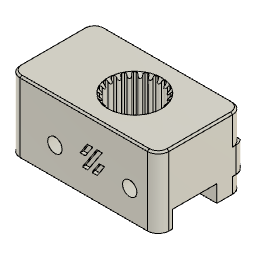
nozzle_probe_ldo (Autodesk Fusion 360 design; units mm, degrees)
Autodesk Fusion 360 part; units mm, degrees
sketch "Sketch1" plane through (0, 0, 0) normal (0, 0, 1) x (1, 0, 0)
  line L0 (17.5, 10) -> (-17.5, 10)
  line L1 (-17.5, 10) -> (-17.5, -10)
  line L2 (-17.5, -10) -> (17.5, -10)
  line L3 (17.5, -10) -> (17.5, 10)
  line L4 (17.5, 10) -> (-17.5, -10) construction
  line L5 (-17.5, 10) -> (17.5, -10) construction
  dimension "d5" = 35
  dimension "d6" = 20
  constraint horizontal L0
  constraint perpendicular L0 L1
  constraint parallel L0 L2
  constraint parallel L1 L3
  constraint coincident L4 origin
  constraint coincident L5 origin
  measures "d5" distance of L0.start L0.end
  measures "d6" distance of L0.start L2.end
extrude "Extrude1" add sketch "Sketch1" against normal blind 16.6
sketch "Sketch2" plane through (0, 0, 0) normal (0, 0, 1) x (-1, 0, 0)
  line L0 (-17.5, 10) -> (-17.5, -10)
  line L1 (-17.5, -10) -> (17.5, -10)
  line L2 (17.5, -10) -> (17.5, 10)
  line L3 (17.5, 10) -> (-17.5, 10)
  circle A0 centre (0, 0) radius 7.61 construction
  arc A1 (5.0953, -3.0231) -> (4.4497, -3.9118) centre (4.7489, -3.4503) ccw construction
  arc A2 (5.0953, -3.0231) -> (5.3358, -2.9768) centre (5.1961, -2.8988) ccw construction
  arc A3 (5.3358, -2.9768) -> (5.5446, -2.5671) centre (0, 0) ccw construction
  arc A4 (5.5446, -2.5671) -> (5.4407, -2.3453) centre (5.3994, -2.4999) ccw construction
  arc A5 (5.7801, -1.3006) -> (5.4407, -2.3453) centre (5.5827, -1.8139) ccw construction
  arc A6 (5.7801, -1.3006) -> (5.9945, -1.1822) centre (5.8376, -1.1512) ccw construction
  arc A7 (5.9945, -1.1822) -> (6.0665, -0.7281) centre (0, 0) ccw construction
  arc A8 (6.0665, -0.7281) -> (5.8991, -0.5492) centre (5.9076, -0.709) ccw construction
  arc A9 (5.8991, 0.5492) -> (5.8991, -0.5492) centre (5.87, 0) ccw construction
  arc A10 (5.8991, 0.5492) -> (6.0665, 0.7281) centre (5.9076, 0.709) ccw construction
  arc A11 (6.0665, 0.7281) -> (5.9945, 1.1822) centre (0, 0) ccw construction
  arc A12 (5.9945, 1.1822) -> (5.7801, 1.3006) centre (5.8376, 1.1512) ccw construction
  arc A13 (5.4407, 2.3453) -> (5.7801, 1.3006) centre (5.5827, 1.8139) ccw construction
  arc A14 (5.4407, 2.3453) -> (5.5446, 2.5671) centre (5.3994, 2.4999) ccw construction
  arc A15 (5.5446, 2.5671) -> (5.3358, 2.9768) centre (0, 0) ccw construction
  arc A16 (5.3358, 2.9768) -> (5.0953, 3.0231) centre (5.1961, 2.8988) ccw construction
  arc A17 (4.4497, 3.9118) -> (5.0953, 3.0231) centre (4.7489, 3.4503) ccw construction
  arc A18 (4.4497, 3.9118) -> (4.4799, 4.1548) centre (4.3626, 4.046) ccw construction
  arc A19 (4.4799, 4.1548) -> (4.1548, 4.4799) centre (0, 0) ccw construction
  arc A20 (4.1548, 4.4799) -> (3.9118, 4.4497) centre (4.046, 4.3626) ccw construction
  arc A21 (3.0231, 5.0953) -> (3.9118, 4.4497) centre (3.4503, 4.7489) ccw construction
  arc A22 (3.0231, 5.0953) -> (2.9768, 5.3358) centre (2.8988, 5.1961) ccw construction
  arc A23 (2.9768, 5.3358) -> (2.5671, 5.5446) centre (0, 0) ccw construction
  arc A24 (2.5671, 5.5446) -> (2.3453, 5.4407) centre (2.4999, 5.3994) ccw construction
  arc A25 (1.3006, 5.7801) -> (2.3453, 5.4407) centre (1.8139, 5.5827) ccw construction
  arc A26 (1.3006, 5.7801) -> (1.1822, 5.9945) centre (1.1512, 5.8376) ccw construction
  arc A27 (1.1822, 5.9945) -> (0.7281, 6.0665) centre (0, 0) ccw construction
  arc A28 (0.7281, 6.0665) -> (0.5492, 5.8991) centre (0.709, 5.9076) ccw construction
  arc A29 (-0.5492, 5.8991) -> (0.5492, 5.8991) centre (0, 5.87) ccw construction
  arc A30 (-0.5492, 5.8991) -> (-0.7281, 6.0665) centre (-0.709, 5.9076) ccw construction
  arc A31 (-0.7281, 6.0665) -> (-1.1822, 5.9945) centre (0, 0) ccw construction
  arc A32 (-1.1822, 5.9945) -> (-1.3006, 5.7801) centre (-1.1512, 5.8376) ccw construction
  arc A33 (-2.3453, 5.4407) -> (-1.3006, 5.7801) centre (-1.8139, 5.5827) ccw construction
  arc A34 (-2.3453, 5.4407) -> (-2.5671, 5.5446) centre (-2.4999, 5.3994) ccw construction
  arc A35 (-2.5671, 5.5446) -> (-2.9768, 5.3358) centre (0, 0) ccw construction
  arc A36 (-2.9768, 5.3358) -> (-3.0231, 5.0953) centre (-2.8988, 5.1961) ccw construction
  arc A37 (-3.9118, 4.4497) -> (-3.0231, 5.0953) centre (-3.4503, 4.7489) ccw construction
  arc A38 (-3.9118, 4.4497) -> (-4.1548, 4.4799) centre (-4.046, 4.3626) ccw construction
  arc A39 (-4.1548, 4.4799) -> (-4.4799, 4.1548) centre (0, 0) ccw construction
  arc A40 (-4.4799, 4.1548) -> (-4.4497, 3.9118) centre (-4.3626, 4.046) ccw construction
  arc A41 (-5.0953, 3.0231) -> (-4.4497, 3.9118) centre (-4.7489, 3.4503) ccw construction
  arc A42 (-5.0953, 3.0231) -> (-5.3358, 2.9768) centre (-5.1961, 2.8988) ccw construction
  arc A43 (-5.3358, 2.9768) -> (-5.5446, 2.5671) centre (0, 0) ccw construction
  arc A44 (-5.5446, 2.5671) -> (-5.4407, 2.3453) centre (-5.3994, 2.4999) ccw construction
  arc A45 (-5.7801, 1.3006) -> (-5.4407, 2.3453) centre (-5.5827, 1.8139) ccw construction
  arc A46 (-5.7801, 1.3006) -> (-5.9945, 1.1822) centre (-5.8376, 1.1512) ccw construction
  arc A47 (-5.9945, 1.1822) -> (-6.0665, 0.7281) centre (0, 0) ccw construction
  arc A48 (-6.0665, 0.7281) -> (-5.8991, 0.5492) centre (-5.9076, 0.709) ccw construction
  arc A49 (-5.8991, -0.5492) -> (-5.8991, 0.5492) centre (-5.87, 0) ccw construction
  arc A50 (-5.8991, -0.5492) -> (-6.0665, -0.7281) centre (-5.9076, -0.709) ccw construction
  arc A51 (-6.0665, -0.7281) -> (-5.9945, -1.1822) centre (0, 0) ccw construction
  arc A52 (-5.9945, -1.1822) -> (-5.7801, -1.3006) centre (-5.8376, -1.1512) ccw construction
  arc A53 (-5.4407, -2.3453) -> (-5.7801, -1.3006) centre (-5.5827, -1.8139) ccw construction
  arc A54 (-5.4407, -2.3453) -> (-5.5446, -2.5671) centre (-5.3994, -2.4999) ccw construction
  arc A55 (-5.5446, -2.5671) -> (-5.3358, -2.9768) centre (0, 0) ccw construction
  arc A56 (-5.3358, -2.9768) -> (-5.0953, -3.0231) centre (-5.1961, -2.8988) ccw construction
  arc A57 (-4.4497, -3.9118) -> (-5.0953, -3.0231) centre (-4.7489, -3.4503) ccw construction
  arc A58 (-4.4497, -3.9118) -> (-4.4799, -4.1548) centre (-4.3626, -4.046) ccw construction
  arc A59 (-4.4799, -4.1548) -> (-4.1548, -4.4799) centre (0, 0) ccw construction
  arc A60 (-4.1548, -4.4799) -> (-3.9118, -4.4497) centre (-4.046, -4.3626) ccw construction
  arc A61 (-3.0231, -5.0953) -> (-3.9118, -4.4497) centre (-3.4503, -4.7489) ccw construction
  arc A62 (-3.0231, -5.0953) -> (-2.9768, -5.3358) centre (-2.8988, -5.1961) ccw construction
  arc A63 (-2.9768, -5.3358) -> (-2.5671, -5.5446) centre (0, 0) ccw construction
  arc A64 (-2.5671, -5.5446) -> (-2.3453, -5.4407) centre (-2.4999, -5.3994) ccw construction
  arc A65 (-1.3006, -5.7801) -> (-2.3453, -5.4407) centre (-1.8139, -5.5827) ccw construction
  arc A66 (-1.3006, -5.7801) -> (-1.1822, -5.9945) centre (-1.1512, -5.8376) ccw construction
  arc A67 (-1.1822, -5.9945) -> (-0.7281, -6.0665) centre (0, 0) ccw construction
  arc A68 (-0.7281, -6.0665) -> (-0.5492, -5.8991) centre (-0.709, -5.9076) ccw construction
  arc A69 (0.5492, -5.8991) -> (-0.5492, -5.8991) centre (0, -5.87) ccw construction
  arc A70 (0.5492, -5.8991) -> (0.7281, -6.0665) centre (0.709, -5.9076) ccw construction
  arc A71 (0.7281, -6.0665) -> (1.1822, -5.9945) centre (0, 0) ccw construction
  arc A72 (1.1822, -5.9945) -> (1.3006, -5.7801) centre (1.1512, -5.8376) ccw construction
  arc A73 (2.3453, -5.4407) -> (1.3006, -5.7801) centre (1.8139, -5.5827) ccw construction
  arc A74 (2.3453, -5.4407) -> (2.5671, -5.5446) centre (2.4999, -5.3994) ccw construction
  arc A75 (2.5671, -5.5446) -> (2.9768, -5.3358) centre (0, 0) ccw construction
  arc A76 (2.9768, -5.3358) -> (3.0231, -5.0953) centre (2.8988, -5.1961) ccw construction
  arc A77 (3.9118, -4.4497) -> (3.0231, -5.0953) centre (3.4503, -4.7489) ccw construction
  arc A78 (3.9118, -4.4497) -> (4.1548, -4.4799) centre (4.046, -4.3626) ccw construction
  arc A79 (4.1548, -4.4799) -> (4.4799, -4.1548) centre (0, 0) ccw construction
  arc A80 (4.4799, -4.1548) -> (4.4497, -3.9118) centre (4.3626, -4.046) ccw construction
  arc A81 (-2.6301, -5.6807) -> (-2.2004, -5.4794) centre (-2.4999, -5.3994) ccw
  arc A82 (-1.4406, -5.7263) -> (-2.2004, -5.4794) centre (-1.8139, -5.5827) ccw
  arc A83 (-1.4406, -5.7263) -> (-1.2112, -6.1417) centre (-1.1512, -5.8376) ccw
  arc A84 (-1.2112, -6.1417) -> (-0.7459, -6.2154) centre (0, 0) ccw
  arc A85 (-0.7459, -6.2154) -> (-0.3994, -5.8912) centre (-0.709, -5.9076) ccw
  arc A86 (0.3994, -5.8912) -> (-0.3994, -5.8912) centre (0, -5.87) ccw
  arc A87 (0.3994, -5.8912) -> (0.7459, -6.2154) centre (0.709, -5.9076) ccw
  arc A88 (0.7459, -6.2154) -> (1.2112, -6.1417) centre (0, 0) ccw
  arc A89 (1.2112, -6.1417) -> (1.4406, -5.7263) centre (1.1512, -5.8376) ccw
  arc A90 (2.2004, -5.4794) -> (1.4406, -5.7263) centre (1.8139, -5.5827) ccw
  arc A91 (2.2004, -5.4794) -> (2.6301, -5.6807) centre (2.4999, -5.3994) ccw
  arc A92 (2.6301, -5.6807) -> (3.0498, -5.4668) centre (0, 0) ccw
  arc A93 (3.0498, -5.4668) -> (3.1396, -5.0009) centre (2.8988, -5.1961) ccw
  arc A94 (3.7859, -4.5313) -> (3.1396, -5.0009) centre (3.4503, -4.7489) ccw
  arc A95 (3.7859, -4.5313) -> (4.2568, -4.5899) centre (4.046, -4.3626) ccw
  arc A96 (4.2568, -4.5899) -> (4.5899, -4.2568) centre (0, 0) ccw
  arc A97 (4.5899, -4.2568) -> (4.5313, -3.7859) centre (4.3626, -4.046) ccw
  arc A98 (5.0009, -3.1396) -> (4.5313, -3.7859) centre (4.7489, -3.4503) ccw
  arc A99 (5.0009, -3.1396) -> (5.4668, -3.0498) centre (5.1961, -2.8988) ccw
  arc A100 (5.4668, -3.0498) -> (5.6807, -2.6301) centre (0, 0) ccw
  arc A101 (5.6807, -2.6301) -> (5.4794, -2.2004) centre (5.3994, -2.4999) ccw
  arc A102 (5.7263, -1.4406) -> (5.4794, -2.2004) centre (5.5827, -1.8139) ccw
  arc A103 (5.7263, -1.4406) -> (6.1417, -1.2112) centre (5.8376, -1.1512) ccw
  arc A104 (6.1417, -1.2112) -> (6.2154, -0.7459) centre (0, 0) ccw
  arc A105 (6.2154, -0.7459) -> (5.8912, -0.3994) centre (5.9076, -0.709) ccw
  arc A106 (5.8912, 0.3994) -> (5.8912, -0.3994) centre (5.87, 0) ccw
  arc A107 (5.8912, 0.3994) -> (6.2154, 0.7459) centre (5.9076, 0.709) ccw
  arc A108 (6.2154, 0.7459) -> (6.1417, 1.2112) centre (0, 0) ccw
  arc A109 (6.1417, 1.2112) -> (5.7263, 1.4406) centre (5.8376, 1.1512) ccw
  arc A110 (5.4794, 2.2004) -> (5.7263, 1.4406) centre (5.5827, 1.8139) ccw
  arc A111 (5.4794, 2.2004) -> (5.6807, 2.6301) centre (5.3994, 2.4999) ccw
  arc A112 (5.6807, 2.6301) -> (5.4668, 3.0498) centre (0, 0) ccw
  arc A113 (5.4668, 3.0498) -> (5.0009, 3.1396) centre (5.1961, 2.8988) ccw
  arc A114 (4.5313, 3.7859) -> (5.0009, 3.1396) centre (4.7489, 3.4503) ccw
  arc A115 (4.5313, 3.7859) -> (4.5899, 4.2568) centre (4.3626, 4.046) ccw
  arc A116 (4.5899, 4.2568) -> (4.2568, 4.5899) centre (0, 0) ccw
  arc A117 (4.2568, 4.5899) -> (3.7859, 4.5313) centre (4.046, 4.3626) ccw
  arc A118 (3.1396, 5.0009) -> (3.7859, 4.5313) centre (3.4503, 4.7489) ccw
  arc A119 (3.1396, 5.0009) -> (3.0498, 5.4668) centre (2.8988, 5.1961) ccw
  arc A120 (3.0498, 5.4668) -> (2.6301, 5.6807) centre (0, 0) ccw
  arc A121 (2.6301, 5.6807) -> (2.2004, 5.4794) centre (2.4999, 5.3994) ccw
  arc A122 (1.4406, 5.7263) -> (2.2004, 5.4794) centre (1.8139, 5.5827) ccw
  arc A123 (1.4406, 5.7263) -> (1.2112, 6.1417) centre (1.1512, 5.8376) ccw
  arc A124 (1.2112, 6.1417) -> (0.7459, 6.2154) centre (0, 0) ccw
  arc A125 (0.7459, 6.2154) -> (0.3994, 5.8912) centre (0.709, 5.9076) ccw
  arc A126 (-0.3994, 5.8912) -> (0.3994, 5.8912) centre (0, 5.87) ccw
  arc A127 (-0.3994, 5.8912) -> (-0.7459, 6.2154) centre (-0.709, 5.9076) ccw
  arc A128 (-0.7459, 6.2154) -> (-1.2112, 6.1417) centre (0, 0) ccw
  arc A129 (-1.2112, 6.1417) -> (-1.4406, 5.7263) centre (-1.1512, 5.8376) ccw
  arc A130 (-2.2004, 5.4794) -> (-1.4406, 5.7263) centre (-1.8139, 5.5827) ccw
  arc A131 (-2.2004, 5.4794) -> (-2.6301, 5.6807) centre (-2.4999, 5.3994) ccw
  arc A132 (-2.6301, 5.6807) -> (-3.0498, 5.4668) centre (0, 0) ccw
  arc A133 (-3.0498, 5.4668) -> (-3.1396, 5.0009) centre (-2.8988, 5.1961) ccw
  arc A134 (-3.7859, 4.5313) -> (-3.1396, 5.0009) centre (-3.4503, 4.7489) ccw
  arc A135 (-3.7859, 4.5313) -> (-4.2568, 4.5899) centre (-4.046, 4.3626) ccw
  arc A136 (-4.2568, 4.5899) -> (-4.5899, 4.2568) centre (0, 0) ccw
  arc A137 (-4.5899, 4.2568) -> (-4.5313, 3.7859) centre (-4.3626, 4.046) ccw
  arc A138 (-5.0009, 3.1396) -> (-4.5313, 3.7859) centre (-4.7489, 3.4503) ccw
  arc A139 (-5.0009, 3.1396) -> (-5.4668, 3.0498) centre (-5.1961, 2.8988) ccw
  arc A140 (-5.4668, 3.0498) -> (-5.6807, 2.6301) centre (0, 0) ccw
  arc A141 (-5.6807, 2.6301) -> (-5.4794, 2.2004) centre (-5.3994, 2.4999) ccw
  arc A142 (-5.7263, 1.4406) -> (-5.4794, 2.2004) centre (-5.5827, 1.8139) ccw
  arc A143 (-5.7263, 1.4406) -> (-6.1417, 1.2112) centre (-5.8376, 1.1512) ccw
  arc A144 (-6.1417, 1.2112) -> (-6.2154, 0.7459) centre (0, 0) ccw
  arc A145 (-6.2154, 0.7459) -> (-5.8912, 0.3994) centre (-5.9076, 0.709) ccw
  arc A146 (-5.8912, -0.3994) -> (-5.8912, 0.3994) centre (-5.87, 0) ccw
  arc A147 (-5.8912, -0.3994) -> (-6.2154, -0.7459) centre (-5.9076, -0.709) ccw
  arc A148 (-6.2154, -0.7459) -> (-6.1417, -1.2112) centre (0, 0) ccw
  arc A149 (-6.1417, -1.2112) -> (-5.7263, -1.4406) centre (-5.8376, -1.1512) ccw
  arc A150 (-5.4794, -2.2004) -> (-5.7263, -1.4406) centre (-5.5827, -1.8139) ccw
  arc A151 (-5.4794, -2.2004) -> (-5.6807, -2.6301) centre (-5.3994, -2.4999) ccw
  arc A152 (-5.6807, -2.6301) -> (-5.4668, -3.0498) centre (0, 0) ccw
  arc A153 (-5.4668, -3.0498) -> (-5.0009, -3.1396) centre (-5.1961, -2.8988) ccw
  arc A154 (-4.5313, -3.7859) -> (-5.0009, -3.1396) centre (-4.7489, -3.4503) ccw
  arc A155 (-4.5313, -3.7859) -> (-4.5899, -4.2568) centre (-4.3626, -4.046) ccw
  arc A156 (-4.5899, -4.2568) -> (-4.2568, -4.5899) centre (0, 0) ccw
  arc A157 (-4.2568, -4.5899) -> (-3.7859, -4.5313) centre (-4.046, -4.3626) ccw
  arc A158 (-3.1396, -5.0009) -> (-3.7859, -4.5313) centre (-3.4503, -4.7489) ccw
  arc A159 (-3.1396, -5.0009) -> (-3.0498, -5.4668) centre (-2.8988, -5.1961) ccw
  arc A160 (-3.0498, -5.4668) -> (-2.6301, -5.6807) centre (0, 0) ccw
  circle A161 centre (0, 0) radius 5.32
  dimension "d9" = -0.15
  constraint concentric A0 A161
  constraint tangent A61 A161
  measures "d56" distance of A20.end
extrude "Extrude3" cut sketch "Sketch2" against normal blind 5 contours A161
chamfer "Chamfer1" distance 1 angle 45 1 edges at (4.96, -1.9238, 0)
extrude "Extrude2" cut sketch "Sketch2" against normal blind 9 contours A81 A82 A83 A84 A85 A86 A87 A88 A89 A90 A91 A92 A93 A94 A95 A96 A97 A98 A99 A100 A101 A102 A103 A104 A105 A106 A107 A108 A109 A110 A111 A112 A113 A114 A115 A116 A117 A118 A119 A120 A121 A122 A123 A124 A125 A126 A127 A128 A129 A130 A131 A132 A133 A134 A135 A136 A137 A138 A139 A140 A141 A142 A143 A144 A145 A146 A147 A148 A149 A150 A151 A152 A153 A154 A155 A156 A157 A158 A159 A160 | A161
sketch "Sketch3" plane through (0, -10, 0) normal (0, -1, 0) x (1, 0, 0)
  line L0 (17.5, 0) -> (-17.5, 0)
  line L1 (-17.5, 0) -> (-17.5, -16.6)
  line L2 (-17.5, -16.6) -> (17.5, -16.6)
  line L3 (17.5, -16.6) -> (17.5, 0)
  line L4 (-17.5, -7) -> (17.5, -7)
  line L5 (17.5, -7) -> (17.5, -13)
  line L6 (17.5, -13) -> (-17.5, -13)
  line L7 (-17.5, -13) -> (-17.5, -7)
  dimension "d15" = 7
  dimension "d16" = 6
  constraint horizontal L4
  constraint vertical L5
  constraint horizontal L6
  constraint vertical L7
  constraint coincident L3 L5.end
  constraint coincident L1 L4.start
  measures "d15" distance of L0 L4
  measures "d16" distance of L4 L6
extrude "Extrude4" add sketch "Sketch3" against normal blind 0.8 from surface at -20 contours L1 L3 L4 L5 L6 L7
sketch "Sketch4" plane through (0, 10.8, 0) normal (0, 1, 0) x (1, 0, 0)
  line L0 (17.5, 13) -> (-17.5, 13)
  line L1 (17.5, 7) -> (17.5, 13)
  line L2 (-17.5, 7) -> (17.5, 7)
  line L3 (-17.5, 13) -> (-17.5, 7)
  line L4 (0, 7) -> (0, 13) construction
  line L5 (-8.8, 10) -> (8.8, 10) construction
  circle A0 centre (-8.8, 10) radius 1.7
  circle A1 centre (8.8, 10) radius 1.7
  dimension "d19" = 17.6
  dimension "d20" = 3.4
  dimension "d21" = 3.4
  constraint midpoint L2 L4.start
  constraint midpoint L0 L4.end
  constraint perpendicular L3 L5
  constraint midpoint L4 L5
  constraint coincident L5.start A0.centre
  constraint coincident L5.end A1.centre
  measures "d19" distance of L5.start L5.end
  measures "d20" diameter of A0
  measures "d21" diameter of A1
extrude "Extrude5" cut sketch "Sketch4" against normal through all contours A0 | A1
sketch "Sketch5" plane through (0, 0, -16.6) normal (0, 0, -1) x (1, 0, 0)
  line L0 (17.5, -10) -> (17.5, 10)
  line L1 (17.5, 10) -> (-17.5, 10)
  line L2 (-17.5, 10) -> (-17.5, -10)
  line L3 (-17.5, -10) -> (17.5, -10)
  line L4 (-3.1, 8) -> (3.1, 8)
  line L5 (3.1, 8) -> (3.1, -5.2)
  line L6 (3.1, -5.2) -> (-3.1, -5.2)
  line L7 (-3.1, -5.2) -> (-3.1, 8)
  line L8 (0, -5.2) -> (0, 8) construction
  point P0 (0, 1.4)
  dimension "d23" = 6.2
  dimension "d24" = 13.2
  dimension "d25" = 1.4
  constraint horizontal L4
  constraint vertical L5
  constraint horizontal L6
  constraint vertical L7
  constraint midpoint L6 L8.start
  constraint midpoint L4 L8.end
  constraint coincident origin L8
  constraint midpoint L8 P0
  measures "d23" distance of L5.end L6.end
  measures "d24" distance of L4.start L6.end
  measures "d25" distance of origin P0
extrude "Extrude6" cut sketch "Sketch5" against normal up to surface (6.8 mm away) contours L4 L5 L6 L7
sketch "Sketch6" plane through (0, 0, -9.8) normal (0, 0, -1) x (1, 0, 0)
  line L0 (3.1, -5.2) -> (3.1, 8)
  line L1 (3.1, 8) -> (-3.1, 8)
  line L2 (-3.1, 8) -> (-3.1, -5.2)
  line L3 (-3.1, -5.2) -> (3.1, -5.2)
  line L4 (-3.1, 4.8) -> (3.1, 4.8)
  dimension "d28" = 3.2
  constraint coincident L2 L4.start
  constraint coincident L0 L4.end
  constraint perpendicular L0 L4
  measures "d28" distance of L0.end L4.end
extrude "Extrude7" cut sketch "Sketch6" against normal up to surface (0.8 mm away) contours L0 L2 L3 L4
sketch "Sketch7" plane through (-17.5, 0, 0) normal (-1, 0, 0) x (0, -1, 0)
  line L0 (10, 0) -> (-10, 0)
  line L1 (-10, 0) -> (-10, -7)
  line L2 (-10, -16.6) -> (10, -16.6)
  line L3 (-10.8, -13) -> (-10, -13)
  line L4 (-10.8, -7) -> (-10.8, -13)
  line L5 (-10, -7) -> (-10.8, -7)
  line L6 (10, -16.6) -> (10, 0)
  line L7 (-5.2, -16.6) -> (5.2, -16.6)
  line L8 (5.2, -16.6) -> (5.2, -10.4)
  line L9 (5.2, -10.4) -> (-5.2, -10.4)
  line L10 (-5.2, -10.4) -> (-5.2, -16.6)
  line L11 (-1.775, -10.4) -> (1.775, -10.4)
  line L12 (1.775, -10.4) -> (1.775, -7.6)
  line L13 (1.775, -7.6) -> (-1.775, -7.6)
  line L14 (-1.775, -7.6) -> (-1.775, -10.4)
  line L15 (-10, -13) -> (-10, -16.6)
  dimension "d31" = 6.2
  dimension "d32" = 10.4
  dimension "d33" = 3.55
  dimension "d34" = 2.8
  constraint horizontal L7
  constraint vertical L8
  constraint horizontal L9
  constraint vertical L10
  constraint coincident L2 L7.start
  constraint midpoint L2 L7
  constraint horizontal L11
  constraint vertical L12
  constraint horizontal L13
  constraint vertical L14
  constraint coincident L9 L11.start
  constraint midpoint L9 L11
  measures "d31" distance of L7.end L8.end
  measures "d32" distance of L8.end L9.end
  measures "d33" distance of L12.end L13.end
  measures "d34" distance of L11.end L12.end
extrude "Extrude8" cut sketch "Sketch7" against normal up to surface (5.4 mm away) contours L2 L7 L8 L9 L10 L11 | L9 L11 L12 L13 L14
extrude "Extrude9" add 1 faces at (-17.5, 0.5917, -2.5333) along direction (-1, 0, 0) blind 2
sketch "Sketch8" plane through (0, 0, -16.6) normal (0, 0, -1) x (1, 0, 0)
  line L0 (-12.1, -5.2) -> (-19.5, -5.2)
  line L1 (-19.5, -5.2) -> (-19.5, -10)
  line L2 (-19.5, -10) -> (17.5, -10)
  line L3 (17.5, -10) -> (17.5, 10)
  line L4 (17.5, 10) -> (-19.5, 10)
  line L5 (-19.5, 10) -> (-19.5, 5.2)
  line L6 (-19.5, 5.2) -> (-12.1, 5.2)
  line L7 (-12.1, 5.2) -> (-12.1, -5.2)
  line L8 (-3.1, -5.2) -> (-3.1, 8)
  line L9 (-3.1, 8) -> (3.1, 8)
  line L10 (3.1, 8) -> (3.1, -5.2)
  line L11 (3.1, -5.2) -> (-3.1, -5.2)
  line L12 (3.1, 6.6) -> (17.5, 6.6)
  line L13 (17.5, 6.6) -> (17.5, -3.8)
  line L14 (17.5, -3.8) -> (3.1, -3.8)
  line L15 (3.1, -3.8) -> (3.1, 6.6)
  dimension "d39" = 10.4
  constraint horizontal L12
  constraint vertical L13
  constraint horizontal L14
  constraint vertical L15
  constraint coincident L3 L13.end
  constraint coincident L10 L12.start
  constraint midpoint L10 L15
  measures "d39" distance of L12.end L13.end
extrude "Extrude10" cut sketch "Sketch8" against normal blind 4 contours L3 L10 L12 L13 L14 L15
sketch "Sketch9" plane through (-3.1, 0, 0) normal (1, 0, 0) x (0, 1, 0)
  line L0 (-4.8, -9.8) -> (-8, -9.8)
  line L1 (-8, -9.8) -> (-8, -16.6)
  line L2 (-8, -16.6) -> (5.2, -16.6)
  line L3 (5.2, -16.6) -> (5.2, -9)
  line L4 (5.2, -9) -> (4.942, -9)
  line L5 (4.942, -9) -> (4.5558, -9)
  line L6 (4.5558, -9) -> (-4.5558, -9)
  line L7 (-4.5558, -9) -> (-4.8, -9)
  line L8 (-4.8, -9) -> (-4.8, -9.8)
  circle A0 centre (-4.65, -14.8) radius 0.8
  circle A1 centre (1.85, -14.8) radius 0.8
  line L9 (1.85, -14.8) -> (-4.65, -14.8) construction
  line L10 (-1.4, -16.6) -> (-1.4, -14.8) construction
  dimension "d42" = 6.5
  dimension "d43" = 1.6
  dimension "d44" = 5
  constraint coincident A1.centre L9.start
  constraint coincident A0.centre L9.end
  constraint horizontal L9
  constraint equal A0 A1
  constraint midpoint L2 L10.start
  constraint perpendicular L2 L10
  constraint midpoint L9 L10.end
  measures "d42" distance of A1.centre A0.centre
  measures "d43" diameter of A1
  measures "d44" vertical distance of L0.start A0.centre
extrude "Extrude11" cut sketch "Sketch9" against normal blind 4.5 contours A0 | A1
extrude "Extrude12" cut 1 faces at (17.5, 1.2667, -4.2) along direction (-1, 0, 0) blind 2
sketch "Sketch10" plane through (0, -10, 0) normal (0, -1, 0) x (1, 0, 0)
  line L0 (15.5, -16.6) -> (15.5, 0)
  line L1 (15.5, 0) -> (-19.5, 0)
  line L2 (-19.5, 0) -> (-19.5, -16.6)
  line L3 (-19.5, -16.6) -> (15.5, -16.6)
  circle A0 centre (-8.8, -10) radius 1.7
  circle A1 centre (8.8, -10) radius 1.7
  line L4 (1.077, -6) -> (-2.327, -11.182)
  line L5 (-2.327, -11.182) -> (-1.077, -11.182)
  line L6 (-1.077, -11.182) -> (2.327, -6)
  line L7 (1.077, -6) -> (2.327, -6)
  line L8 (-0.625, -8.591) -> (0.625, -8.591) construction
  line L9 (0, 0) -> (0, -16.6) construction
  line L10 (-0.077, -11.182) -> (1.173, -11.182)
  line L11 (-0.077, -11.182) -> (1.625, -8.591)
  line L12 (-1.077, -11.182) -> (-0.077, -11.182) construction
  line L13 (0.625, -8.591) -> (1.625, -8.591) construction
  line L14 (1.173, -11.182) -> (2.875, -8.591)
  line L15 (1.625, -8.591) -> (2.875, -8.591)
  line L16 (-0.625, -8.591) -> (-1.625, -8.591) construction
  line L17 (-1.625, -8.591) -> (-2.875, -8.591)
  line L18 (-1.625, -8.591) -> (0.077, -6)
  line L19 (1.077, -6) -> (0.077, -6) construction
  line L20 (-2.875, -8.591) -> (-1.173, -6)
  line L21 (0.077, -6) -> (-1.173, -6)
  point P0 (-0.625, -8.591)
  point P1 (0.625, -8.591)
  point P2 (0, -8.591)
  dimension "d50" = 1.25
  dimension "d51" = 6.2
  dimension "d52" = 56.7
  dimension "d56" = 1
  dimension "d57" = 1
  dimension "d60" = 6
  constraint midpoint L4 P0
  constraint horizontal L5
  constraint parallel L4 L6
  constraint equal L4 L6
  constraint midpoint L6 P1
  constraint coincident P0 L8.start
  constraint coincident P1 L8.end
  constraint coincident L9.start origin
  constraint coincident L3 L9.end
  constraint perpendicular L3 L9
  constraint midpoint L8 P2
  constraint coincident L9 P2
  constraint perpendicular L9 L10
  constraint equal L5 L10
  constraint parallel L6 L11
  constraint parallel L5 L12
  constraint coincident L10.start L11.start
  constraint horizontal L13
  constraint coincident L11.end L13.end
  constraint parallel L11 L14
  constraint equal L11 L14
  constraint perpendicular L9 L16
  constraint parallel L16 L17
  constraint parallel L7 L19
  constraint parallel L4 L18
  constraint coincident L18 L19.end
  constraint equal L18 L20
  constraint parallel L18 L20
  constraint equal L5 L17
  measures "d50" distance of L4.end L5.end
  measures "d51" distance of L4.start L4.end
  measures "d52" angle of L4 L5
  measures "d56" distance of P1 L11.end
  measures "d57" distance of P0 L16.end
  measures "d60" distance of L1 L20.end
extrude "Extrude13" cut sketch "Sketch10" against normal blind 0.8 contours L4 L5 L6 L7 | L10 L11 L14 L15 | L17 L18 L20 L21
fillet "Fillet1" radius 2.5 8 edges at (15.5, -10, -8.3) (-19.5, -10, -8.3) (15.5, 10, -14.8) (15.5, 10, -3.5) (-19.5, 10, -14.8) (-19.5, 10, -3.5) (-19.5, 10.8, -10) (15.5, 10.8, -10)
sketch "Sketch11" plane through (-19.5, 0, 0) normal (-1, 0, 0) x (0, -1, 0)
  line L0 (-8.3, -7) -> (-8.3, -13)
  line L1 (-8.3, -13) -> (-7.5, -13)
  line L2 (-7.5, -13) -> (-7.5, -16.6)
  line L3 (-7.5, -16.6) -> (-5.2, -16.6)
  line L4 (-5.2, -16.6) -> (-5.2, -10.4)
  line L5 (-5.2, -10.4) -> (-1.775, -10.4)
  line L6 (-1.775, -10.4) -> (-1.775, -7.6)
  line L7 (-1.775, -7.6) -> (1.775, -7.6)
  line L8 (1.775, -7.6) -> (1.775, -10.4)
  line L9 (1.775, -10.4) -> (5.2, -10.4)
  line L10 (5.2, -10.4) -> (5.2, -16.6)
  line L11 (5.2, -16.6) -> (7.5, -16.6)
  line L12 (7.5, -16.6) -> (7.5, 0)
  line L13 (7.5, 0) -> (-7.5, 0)
  line L14 (-7.5, 0) -> (-7.5, -7)
  line L15 (-7.5, -7) -> (-8.3, -7)
  line L16 (-10.8, -7) -> (-10.8, -13)
  line L17 (-10.8, -7) -> (-8.3, -7)
  line L18 (-8.3, -13) -> (-10.8, -13)
  line L19 (-10, 0) -> (-10, -7)
  line L20 (-10, -13) -> (-10, -16.6)
  line L21 (-10, -7) -> (-10.8, -7.8)
  line L22 (-10, -13) -> (-10.8, -12.2)
  dimension "d63" = 45
  constraint coincident L19.end L21.start
  constraint coincident L16 L21.end
  constraint coincident L20.start L22.start
  constraint coincident L16 L22.end
  constraint perpendicular L21 L22
  measures "d63" angle of L18 L22
extrude "Extrude14" cut sketch "Sketch11" against normal through all contours L16 L17 L21 | L16 L18 L22
chamfer "Chamfer2" distance 0.4 angle 45 8 edges at (-2, 10, 0) (-18.7678, 9.2678, 0) (-19.5, 0, 0) (-18.7678, -9.2678, 0) (-2, -10, 0) (14.7678, -9.2678, 0) (15.5, 0, 0) (14.7678, 9.2678, 0)
sketch "PCB Layout" plane through (0, 0, -16.6) normal (0, 0, -1) x (1, 0, 0)
  arc A0 (-19.5, -7.5) -> (-17, -10) centre (-17, -7.5) ccw
  line L0 (-17, -10) -> (13, -10)
  arc A1 (13, -10) -> (15.5, -7.5) centre (13, -7.5) ccw
  line L1 (15.5, -7.5) -> (15.5, -3.8)
  line L2 (15.5, -3.8) -> (3.1, -3.8)
  line L3 (3.1, -3.8) -> (3.1, -5.2)
  line L4 (3.1, -5.2) -> (-3.1, -5.2)
  line L5 (-3.1, -5.2) -> (-3.1, 8)
  line L6 (-3.1, 8) -> (3.1, 8)
  line L7 (3.1, 8) -> (3.1, 6.6)
  line L8 (3.1, 6.6) -> (15.5, 6.6)
  line L9 (15.5, 6.6) -> (15.5, 7.5)
  arc A2 (15.5, 7.5) -> (13, 10) centre (13, 7.5) ccw
  line L10 (13, 10) -> (-17, 10)
  arc A3 (-17, 10) -> (-19.5, 7.5) centre (-17, 7.5) ccw
  line L11 (-19.5, 7.5) -> (-19.5, 5.2)
  line L12 (-19.5, 5.2) -> (-12.1, 5.2)
  line L13 (-12.1, 5.2) -> (-12.1, -5.2)
  line L14 (-12.1, -5.2) -> (-19.5, -5.2)
  line L15 (-19.5, -5.2) -> (-19.5, -7.5)
